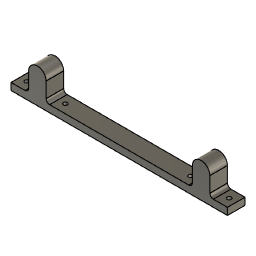
Držáky vedení X v9 (Autodesk Fusion 360 design; units mm, degrees)
Autodesk Fusion 360 part; units mm, degrees
sketch "Bokorys" plane through (0, 0, 0) normal (0, 1, 0) x (1, 0, 0)
  circle A0 centre (0, -22) radius 3
  line L0 (162.5, -6) -> (162.5, 0)
  line L1 (162.5, 0) -> (-22.5, 0)
  line L2 (-22.5, 0) -> (-22.5, -6)
  arc A1 (-7.5, -22) -> (7.5, -22) centre (0, -22) ccw
  line L3 (-22.5, -6) -> (-10.5, -6)
  line L4 (-7.5, -9) -> (-7.5, -22)
  line L5 (7.5, -22) -> (7.5, -9)
  arc A2 (-7.5, -9) -> (-10.5, -6) centre (-10.5, -9) ccw
  arc A3 (10.5, -6) -> (7.5, -9) centre (10.5, -9) ccw
  line L6 (70, 35) -> (70, -50) construction
  arc A4 (132.5, -22) -> (147.5, -22) centre (140, -22) ccw
  circle A5 centre (140, -22) radius 3
  arc A6 (150.5, -6) -> (147.5, -9) centre (150.5, -9) ccw
  line L7 (147.5, -9) -> (147.5, -22)
  line L8 (132.5, -22) -> (132.5, -9)
  arc A7 (132.5, -9) -> (129.5, -6) centre (129.5, -9) ccw
  line L9 (10.5, -6) -> (129.5, -6)
  line L10 (150.5, -6) -> (162.5, -6)
  dimension "d11" = 22
  dimension "d13" = 15
  dimension "d14" = 6
  dimension "d16" = 185
  dimension "d19" = 6
  dimension "d23" = 3
  dimension "d24" = 3
  dimension "d44" = 6
  dimension "d45" = 6
  dimension "d52" = 22.5
  dimension "d53" = 22.5
  dimension "d54" = 92.5
  dimension "d55" = 15
  dimension "d62" = 12.5
  dimension "d72" = 135
  dimension "d73" = 22
  constraint concentric A0 A1
  constraint horizontal L3
  constraint vertical L0
  constraint horizontal L1
  constraint vertical L2
  constraint horizontal L9
  constraint vertical L4
  constraint vertical L5
  constraint tangent L3 A2
  constraint tangent L4 A2
  constraint tangent L5 A3
  constraint tangent A3 L9
  constraint perpendicular L6 L9
  constraint symmetric A0 L6 A5
  constraint symmetric A1 L6 A4
  constraint symmetric A1.start L6 A4.end
  constraint symmetric A1.end L6 A4.start
  constraint symmetric L3.end L6 A6.start
  constraint symmetric L4.start L6 A6.end
  constraint symmetric A2 L6 A6
  constraint symmetric L5.end L6 L8.end
  constraint symmetric A3.start L6 A7.end
  constraint symmetric A3 L6 A7
  constraint collinear L9 L10
  measures "d11" vertical distance of origin A0.centre
  measures "d13" diameter of A1
  measures "d14" diameter of A0
  measures "d16" distance of L0.end L1.end
  measures "d19" vertical distance of origin L2.end
  measures "d23" radius of A2
  measures "d24" radius of A3
  measures "d44" distance of L0.start L0.end
  measures "d45" vertical distance of L2.end L0.end
  measures "d52" horizontal distance of A0.centre L2.end
  measures "d53" distance of origin L1.end
  measures "d54" horizontal distance of L1.end L6.start
  measures "d55" distance of L4 L5
  measures "d73" vertical distance of A0.centre L1.end
extrude "Extrude9" add sketch "Bokorys" along normal blind 15
extrude "Extrude10" add sketch "Bokorys" along normal blind 5 contours A0
extrude "Extrude11" add sketch "Bokorys" along normal blind 5 contours A5
sketch "Sketch6" plane through (0, 0, 0) normal (0, 0, 1) x (1, 0, 0)
  line L0 (-22.5, 0) -> (162.5, 0)
  line L1 (162.5, 0) -> (162.5, 15)
  line L2 (162.5, 15) -> (-22.5, 15)
  line L3 (-22.5, 15) -> (-22.5, 0)
  circle A0 centre (156.5, 7.5) radius 1.75
  line L4 (150.5, 0) -> (162.5, 0)
  circle A1 centre (123.5, 7.5) radius 1.75
  line L5 (70, 42.0713) -> (70, -45) construction
  circle A2 centre (16.5, 7.5) radius 1.75
  circle A3 centre (-16.5, 7.5) radius 1.75
  point P0 (-22.5, 0)
  point P1 (162.5, 15)
  point P2 (162.5, 0)
  point P3 (162.5, 0)
  dimension "d63" = 3.5
  dimension "d64" = 6
  dimension "d65" = 7.5
  dimension "d66" = 3.5
  dimension "d67" = 39
  dimension "d68" = 7.5
  dimension "d69" = 92.5
  constraint horizontal L0
  constraint vertical L1
  constraint horizontal L2
  constraint vertical L3
  constraint coincident P1 L1.end
  constraint coincident P0 L0.start
  constraint vertical L5
  constraint symmetric A0 L5 A3
  constraint symmetric A1 L5 A2
  measures "d63" diameter of A0
  measures "d64" horizontal distance of A0.centre P3
  measures "d65" distance of A0.centre L4
  measures "d66" diameter of A1
  measures "d67" horizontal distance of A1.centre P3
  measures "d68" vertical distance of A1.centre P3
  measures "d69" horizontal distance of P3 L5.end
extrude "Extrude12" cut sketch "Sketch6" along normal blind 15 contours A0 | A1 | A2 | A3
copy_body "Body->Comp1" [suppressed] in component "Úchytka"
named bodies: "Úchytka"
